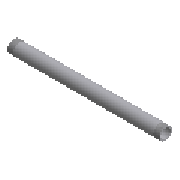
# Autodesk Inventor part: pipipe.1661247839230
Saved by Autodesk Inventor 2023 (Build 270158000, 158)
## iProperties
IsCustomPart: 1
Created: 2022-02-04
Material: Steel, Wrought
Description: Pipe
Document SubType Name: Modeling
Standard: ASME B36.10M
Designer: Mike
Standard Revision: 2004
Standards Organization: ANSI
Language: en-US
Size Designation: 1/2 - Schedule 30 - 4.25
Categories: <MemberInstance><Categories><Category DisplayName="Tube &amp; Pipe" InternalName="4347fa0f-2144-441d-94cd-e3e15c92b736" Mnemonic="TUBEANDPIPE"><CategoryParameter DisplayName="Number of Connections" InternalName="04e9c83a-9e20-4a98-a7e1-e8abe87a2846" Mnemonic="NUM_CONNECTIONS"/><CategoryParameter DisplayName="Angles" InternalName="0e0e4fa4-3bd3-4656-a22e-4e07c8c476f8" Mnemonic="ANGLES"><CategoryParameter DisplayName="Angle" InternalName="9188ad83-1b16-48b4-8b0a-76ce729dafa7" Mnemonic="ANGLE"/></CategoryParameter><CategoryParameter DisplayName="SKey" InternalName="3da84699-049a-4bc2-a65a-6696b77c242f" Mnemonic="SKEY"/><CategoryParameter DisplayName="ISOGEN Description" InternalName="7aa3ba45-b821-4467-8584-f9e6f15f2a7d" Mnemonic="ISOGENDESC"/><CategoryParameter DisplayName="ITEM-CODE" InternalName="99cc3b15-24d9-4d38-aac7-792cfbc57acf" Mnemonic="ITEMCODE"/><CategoryParameter DisplayName="NameOfComponent" InternalName="9c74ad13-48a1-45fe-b0f7-5447561f444a" Mnemonic="NAMEOFCOMPONENT"/><CategoryParameter DisplayName="InLineGroups" InternalName="d60be647-bc43-4c18-a13f-9fe4115f8e64" Mnemonic="INLINEGROUPS"/><Category DisplayName="Conduits" InternalName="0917448a-7f4d-4362-b21b-a60d05e1c56f" Mnemonic="CONDUITS"><CategoryParameter DisplayName="PipeLength" InternalName="84233622-ea40-4b53-b636-458d54f3a9e0" Mnemonic="PL"/><CategoryParameter DisplayName="Connections" InternalName="ef1b9597-584c-4227-9e47-647057e92f71" Mnemonic="PIPE_CONNECTIONS"><CategoryParameter DisplayName="Gender Neutral" InternalName="0135de5f-ee32-4593-8b66-ab45f5df415d" Mnemonic="NEUTRAL"/><CategoryParameter DisplayName="OuterDiameter" InternalName="082ea741-3dcf-4853-908c-481f2491b57d" Mnemonic="OD"/><CategoryParameter DisplayName="MinEngagement [% of MaxEngagement]" InternalName="3e1ca047-d004-446e-8b7d-e3d2ffcfa6ae" Mnemonic="MINENGAGEMENT"/><CategoryParameter DisplayName="FlipDirection" InternalName="6711cd9d-6b7e-47bf-b3fd-37395011a06e" Mnemonic="FLIPDIRECTION"/><CategoryParameter DisplayName="EndTreatment" InternalName="6bdd7eeb-ca9f-479f-914a-a6f58ba02ecf" Mnemonic="ENDTREATMENT"/><CategoryParameter DisplayName="NominalSize" InternalName="8d3dc73b-63e9-4bca-af78-1523b571a978" Mnemonic="NS"/><CategoryParameter DisplayName="InnerDiameter" InternalName="8f0e7e1d-0c1a-450d-a3ea-acf6fdc37b38" Mnemonic="ID"/><CategoryParameter DisplayName="Female" InternalName="91a68ca8-89f8-430e-94a7-98da7f5558a1" Mnemonic="FEMALE"/><CategoryParameter DisplayName="MaxEngagement" InternalName="ca99fb4d-bf82-4017-ae60-624d35c0ac37" Mnemonic="MAXENGAGEMENT"/><CategoryParameter DisplayName="DisplayName" InternalName="eb067ee5-9455-4a40-a436-ea6da7417161" Mnemonic="DISPLAYNAME"/><CategoryParameter DisplayName="Fixed" InternalName="fcf2b1e1-6728-4f9c-9e27-68dda4edbfa5" Mnemonic="FIXED"/><CategoryParameter DisplayName="ScheduleNumber" InternalName="fd9d4457-3734-4b7e-ad1f-37a31a426796" Mnemonic="SN"/></CategoryParameter><CategoryParameter DisplayName="Connections" InternalName="ef1b9597-584c-4227-9e47-647057e92f71" Mnemonic="PIPE_CONNECTIONS"><CategoryParameter DisplayName="Gender Neutral" InternalName="0135de5f-ee32-4593-8b66-ab45f5df415d" Mnemonic="NEUTRAL"/><CategoryParameter DisplayName="OuterDiameter" InternalName="082ea741-3dcf-4853-908c-481f2491b57d" Mnemonic="OD"/><CategoryParameter DisplayName="MinEngagement [% of MaxEngagement]" InternalName="3e1ca047-d004-446e-8b7d-e3d2ffcfa6ae" Mnemonic="MINENGAGEMENT"/><CategoryParameter DisplayName="FlipDirection" InternalName="6711cd9d-6b7e-47bf-b3fd-37395011a06e" Mnemonic="FLIPDIRECTION"/><CategoryParameter DisplayName="EndTreatment" InternalName="6bdd7eeb-ca9f-479f-914a-a6f58ba02ecf" Mnemonic="ENDTREATMENT"/><CategoryParameter DisplayName="NominalSize" InternalName="8d3dc73b-63e9-4bca-af78-1523b571a978" Mnemonic="NS"/><CategoryParameter DisplayName="InnerDiameter" InternalName="8f0e7e1d-0c1a-450d-a3ea-acf6fdc37b38" Mnemonic="ID"/><CategoryParameter DisplayName="Female" InternalName="91a68ca8-89f8-430e-94a7-98da7f5558a1" Mnemonic="FEMALE"/><CategoryParameter DisplayName="MaxEngagement" InternalName="ca99fb4d-bf82-4017-ae60-624d35c0ac37" Mnemonic="MAXENGAGEMENT"/><CategoryParameter DisplayName="DisplayName" InternalName="eb067ee5-9455-4a40-a436-ea6da7417161" Mnemonic="DISPLAYNAME"/><CategoryParameter DisplayName="Fixed" InternalName="fcf2b1e1-6728-4f9c-9e27-68dda4edbfa5" Mnemonic="FIXED"/><CategoryParameter DisplayName="ScheduleNumber" InternalName="fd9d4457-3734-4b7e-ad1f-37a31a426796" Mnemonic="SN"/></CategoryParameter><Category DisplayName="Pipes" InternalName="b7e6be6b-6eb8-4fff-9fa6-a2e6ed0c1528" Mnemonic="PIPES"/></Category></Category><Category DisplayName="DataType" InternalName="23b78d0f-2648-40c6-8793-ca6db495c9e8" Mnemonic="DATATYPE"><CategoryParameter DisplayName="DisplayName" InternalName="05415f3d-3907-474b-a020-eb9d644f4cf3" Mnemonic="DISPLAYNAME"/><CategoryParameter DisplayName="Standard" InternalName="0c0a119c-1e12-4c84-803f-101930972f5e" Mnemonic="STANDARD"/><CategoryParameter DisplayName="Description" InternalName="13903e3d-64b1-4950-80da-f627842ea37f" Mnemonic="DESCRIPTION"/><CategoryParameter DisplayName="Designation" InternalName="2675968c-4ce5-49e0-a4f5-552d29089031" Mnemonic="DESIGNATION"/><CategoryParameter DisplayName="Default Row" InternalName="2af9ec52-faaa-4026-b378-f9fa4afca842" Mnemonic="DEFAULTROW"/><CategoryParameter DisplayName="Folder Name" InternalName="3f06958e-8713-4116-9be7-ed6184ecc97b" Mnemonic="FOLDERNAME"/><CategoryParameter DisplayName="Revision Guid" InternalName="45a75005-10b1-4dfc-8d6d-dfe629f0b93c" Mnemonic="REVISIONGUID"/><CategoryParameter DisplayName="FileName" InternalName="8b46a4cc-9585-4fed-90c3-899f57e09a73" Mnemonic="FILENAME"/><CategoryParameter DisplayName="StdsOrg" InternalName="8f5914e1-4693-403f-8ab5-d37768198c9d" Mnemonic="STDSORG"/><CategoryParameter DisplayName="Family Version" InternalName="914462f6-6e19-4b14-ba84-155b9680b1d0" Mnemonic="FAMILYREVISION"/><CategoryParameter DisplayName="Standard Revision" InternalName="91d5a463-65c2-4fde-b823-3b7fea5e8e17" Mnemonic="STANDARDREVISION"/><CategoryParameter DisplayName="Member Revision" InternalName="a65d44b9-392f-4f4f-857b-e4b3d54996fe" Mnemonic="MEMBERREVISION"/><CategoryParameter DisplayName="ClipFormat" InternalName="bc51e27b-3422-4e78-93ef-cec197ddf230" Mnemonic="CLIPFORMAT"/><CategoryParameter DisplayName="Manufacturer" InternalName="cd6c7a72-a28a-4e50-99a9-2c7f4e13e5ad" Mnemonic="MANUFACTURER"/><CategoryParameter DisplayName="InternalName" InternalName="cf1d0246-76d9-4b4a-8305-fa0409afb5c1" Mnemonic="INTERNALNAME"/><CategoryParameter DisplayName="IsMetric" InternalName="e2385c5b-1ea4-4823-96a8-8de651266ec3" Mnemonic="ISMETRIC"/><Category DisplayName="Part" InternalName="c0e0b642-3bcb-4cc8-9e80-f96d35c4afa4" Mnemonic="PART"><CategoryParameter DisplayName="Part Number" InternalName="016b6077-bfbe-49bd-92c9-d8d59c39c941" Mnemonic="PARTNUMBER"/><CategoryParameter DisplayName="Stock Number" InternalName="4dba7c1c-e26c-444e-836c-b08b433409a8" Mnemonic="STOCKNUMBER"/><CategoryParameter DisplayName="Material Key" InternalName="5c9a8adb-dd2b-4535-b97f-0a94a95fe41f" Mnemonic="MATERIALKEY"/><CategoryParameter DisplayName="Material" InternalName="818a152a-d3c3-49ca-80ee-df7d91421b8e" Mnemonic="MATERIAL"/></Category></Category><Category DisplayName="LegacyMap" InternalName="dfeab48a-acc2-4514-a11c-1b8dc28c3d5f" Mnemonic="LEGACYMAP"><CategoryParameter DisplayName="CatalogID" InternalName="0da51c36-8fd3-4028-86cc-0c9c9e96136a" Mnemonic="CATALOGID"/><CategoryParameter DisplayName="FamilyID" InternalName="1c0b589c-8bbe-4e1e-80cf-07c0de42ac2a" Mnemonic="FAMILYID"/><CategoryParameter DisplayName="MemberID" InternalName="a368ea03-db8a-4d6e-962b-2aa46306b8f5" Mnemonic="MEMBERID"/></Category></Categories><FamilyTemplate Id="ASME B36.10M Pipe with Threaded Ends"><FamilyTemplateParameters><FamilyTemplateParameter ObjectType="kUserParameterObject" ValueType="xs:double" Id="1" ObjectReferenceKey="OD"/><FamilyTemplateParameter ObjectType="kUserParameterObject" ValueType="xs:double" Id="2" ObjectReferenceKey="t"/><FamilyTemplateParameter ObjectType="kUserParameterObject" ValueType="xs:double" Id="3" ObjectReferenceKey="PL"/><FamilyTemplateParameter ObjectType="kUserParameterObject" ValueType="xs:double" Id="4" ObjectReferenceKey="ID"/><FamilyTemplateParameter ObjectType="kUserParameterObject" ValueType="xs:double" Id="5" ObjectReferenceKey="L4"/><FamilyTemplateParameter ObjectType="kUserParameterObject" ValueType="xs:double" Id="6" ObjectReferenceKey="L"/><FamilyTemplateParameter ObjectType="kUserParameterObject" ValueType="xs:double" Id="7" ObjectReferenceKey="L2"/><FamilyTemplateParameter ObjectType="kUserParameterObject" ValueType="xs:double" Id="8" ObjectReferenceKey="D2"/><FamilyTemplateParameter ObjectType="kUserParameterObject" ValueType="xs:string" Id="120" ObjectReferenceKey="Size_Designation"/><FamilyTemplateParameter ObjectType="kUserParameterObject" ValueType="xs:double" Id="126" ObjectReferenceKey="PLmin"/><FamilyTemplateParameter ObjectType="kPropertyObject" ValueType="xs:string" Id="100" ObjectReferenceKey="{32853F0F-3444-11d1-9E93-0060B03C1CA6}" SubObjectId="52"/><FamilyTemplateParameter ObjectType="kPropertyObject" ValueType="xs:string" Id="105" ObjectReferenceKey="{32853F0F-3444-11d1-9E93-0060B03C1CA6}" SubObjectId="5"/><FamilyTemplateParameter ObjectType="kPartComponentDefinitionObject" ValueType="xs:string" Id="110" SubObjectId="Material"/><FamilyTemplateParameter ObjectType="kPropertyObject" ValueType="xs:string" Id="111" ObjectReferenceKey="{32853F0F-3444-11d1-9E93-0060B03C1CA6}" SubObjectId="55"/><FamilyTemplateParameter ObjectType="kThreadFeatureObject" ValueType="xs:structure" Id="300" ObjectReferenceKey="10020000100000000A230000000000008000000000000000" SubObjectId="ThreadInfo"><FamilyTemplateParameter ObjectType="" ValueType="xs:string" Id="301" SubObjectId="ThreadType"/><FamilyTemplateParameter ObjectType="" ValueType="xs:string" Id="302" SubObjectId="NominalDiameter"/></FamilyTemplateParameter><FamilyTemplateParameter ObjectType="kThreadFeatureObject" ValueType="xs:structure" Id="303" ObjectReferenceKey="100200001000000041230000000000008000000000000000" SubObjectId="ThreadInfo"><FamilyTemplateParameter ObjectType="" ValueType="xs:string" Id="304" SubObjectId="ThreadType"/><FamilyTemplateParameter ObjectType="" ValueType="xs:string" Id="305" SubObjectId="NominalDiameter"/></FamilyTemplateParameter></FamilyTemplateParameters></FamilyTemplate><CategoryParameterMap><ParamToTemplateMap><ParamToTemplate CategoryParameter="//CategoryParameter[@InternalName='d60be647-bc43-4c18-a13f-9fe4115f8e64']" ConstantValue="1"/><ParamToTemplate CategoryParameter="//CategoryParameter[@InternalName='04e9c83a-9e20-4a98-a7e1-e8abe87a2846']" ConstantValue="2"/><ParamToTemplate CategoryParameter="//CategoryParameter[@InternalName='0e0e4fa4-3bd3-4656-a22e-4e07c8c476f8']" ConstantValue=""/><ParamToTemplate CategoryParameter="//CategoryParameter[@InternalName='0e0e4fa4-3bd3-4656-a22e-4e07c8c476f8'][1]/CategoryParameter[@InternalName='9188ad83-1b16-48b4-8b0a-76ce729dafa7']" ConstantValue="3.14159265358979"/><ParamToTemplate CategoryParameter="//CategoryParameter[@InternalName='ef1b9597-584c-4227-9e47-647057e92f71'][1]/CategoryParameter[@InternalName='6711cd9d-6b7e-47bf-b3fd-37395011a06e']" ConstantValue="true"/><ParamToTemplate CategoryParameter="//CategoryParameter[@InternalName='ef1b9597-584c-4227-9e47-647057e92f71'][1]/CategoryParameter[@InternalName='eb067ee5-9455-4a40-a436-ea6da7417161']" ConstantValue="Connection1"/><ParamToTemplate CategoryParameter="//CategoryParameter[@InternalName='ef1b9597-584c-4227-9e47-647057e92f71'][1]/CategoryParameter[@InternalName='91a68ca8-89f8-430e-94a7-98da7f5558a1']" ConstantValue="false"/><ParamToTemplate CategoryParameter="//CategoryParameter[@InternalName='ef1b9597-584c-4227-9e47-647057e92f71'][1]/CategoryParameter[@InternalName='6bdd7eeb-ca9f-479f-914a-a6f58ba02ecf']" ConstantValue="Threaded"/><ParamToTemplate CategoryParameter="//CategoryParameter[@InternalName='ef1b9597-584c-4227-9e47-647057e92f71'][1]/CategoryParameter[@InternalName='fcf2b1e1-6728-4f9c-9e27-68dda4edbfa5']" ConstantValue="false"/><ParamToTemplate CategoryParameter="//CategoryParameter[@InternalName='ef1b9597-584c-4227-9e47-647057e92f71'][1]/CategoryParameter[@InternalName='ca99fb4d-bf82-4017-ae60-624d35c0ac37']" ConstantValue="0"/><ParamToTemplate CategoryParameter="//CategoryParameter[@InternalName='ef1b9597-584c-4227-9e47-647057e92f71'][1]/CategoryParameter[@InternalName='3e1ca047-d004-446e-8b7d-e3d2ffcfa6ae']" ConstantValue="20"/><ParamToTemplate CategoryParameter="//CategoryParameter[@InternalName='ef1b9597-584c-4227-9e47-647057e92f71'][2]/CategoryParameter[@InternalName='6711cd9d-6b7e-47bf-b3fd-37395011a06e']" ConstantValue="false"/><ParamToTemplate CategoryParameter="//CategoryParameter[@InternalName='ef1b9597-584c-4227-9e47-647057e92f71'][2]/CategoryParameter[@InternalName='eb067ee5-9455-4a40-a436-ea6da7417161']" ConstantValue="Connection2"/><ParamToTemplate CategoryParameter="//CategoryParameter[@InternalName='ef1b9597-584c-4227-9e47-647057e92f71'][2]/CategoryParameter[@InternalName='91a68ca8-89f8-430e-94a7-98da7f5558a1']" ConstantValue="false"/><ParamToTemplate CategoryParameter="//CategoryParameter[@InternalName='ef1b9597-584c-4227-9e47-647057e92f71'][2]/CategoryParameter[@InternalName='6bdd7eeb-ca9f-479f-914a-a6f58ba02ecf']" ConstantValue="Threaded"/><ParamToTemplate CategoryParameter="//CategoryParameter[@InternalName='ef1b9597-584c-4227-9e47-647057e92f71'][2]/CategoryParameter[@InternalName='fcf2b1e1-6728-4f9c-9e27-68dda4edbfa5']" ConstantValue="false"/><ParamToTemplate CategoryParameter="//CategoryParameter[@InternalName='ef1b9597-584c-4227-9e47-647057e92f71'][2]/CategoryParameter[@InternalName='ca99fb4d-bf82-4017-ae60-624d35c0ac37']" ConstantValue="0"/><ParamToTemplate CategoryParameter="//CategoryParameter[@InternalName='ef1b9597-584c-4227-9e47-647057e92f71'][2]/CategoryParameter[@InternalName='3e1ca047-d004-446e-8b7d-e3d2ffcfa6ae']" ConstantValue="20"/><ParamToTemplate CategoryParameter="//CategoryParameter[@InternalName='05415f3d-3907-474b-a020-eb9d644f4cf3']" ConstantValue="ASME B36.10M Pipe with Threaded Ends"/><ParamToTemplate CategoryParameter="//CategoryParameter[@InternalName='cf1d0246-76d9-4b4a-8305-fa0409afb5c1']" ConstantValue="4a736116-503a-44ad-a922-868ac6b46736"/><ParamToTemplate CategoryParameter="//CategoryParameter[@InternalName='3f06958e-8713-4116-9be7-ed6184ecc97b']" ConstantValue="ASME B36.10M(2)"/><ParamToTemplate CategoryParameter="//CategoryParameter[@InternalName='914462f6-6e19-4b14-ba84-155b9680b1d0']" ConstantValue="10"/><ParamToTemplate CategoryParameter="//CategoryParameter[@InternalName='13903e3d-64b1-4950-80da-f627842ea37f']" ConstantValue="Pipe"/><ParamToTemplate CategoryParameter="//CategoryParameter[@InternalName='8f5914e1-4693-403f-8ab5-d37768198c9d']" ConstantValue="ANSI"/><ParamToTemplate CategoryParameter="//CategoryParameter[@InternalName='0c0a119c-1e12-4c84-803f-101930972f5e']" ConstantValue="ASME B36.10M"/><ParamToTemplate CategoryParameter="//CategoryParameter[@InternalName='cd6c7a72-a28a-4e50-99a9-2c7f4e13e5ad']" TemplateParameter="104"/><ParamToTemplate CategoryParameter="//CategoryParameter[@InternalName='91d5a463-65c2-4fde-b823-3b7fea5e8e17']" ConstantValue="2004"/><ParamToTemplate CategoryParameter="//CategoryParameter[@InternalName='bc51e27b-3422-4e78-93ef-cec197ddf230']" ConstantValue="CF_INVENTOR.STDPARTS"/><ParamToTemplate CategoryParameter="//CategoryParameter[@InternalName='e2385c5b-1ea4-4823-96a8-8de651266ec3']" ConstantValue="false"/><ParamToTemplate CategoryParameter="//CategoryParameter[@InternalName='45a75005-10b1-4dfc-8d6d-dfe629f0b93c']" ConstantValue="1b3bb503-a999-4b6a-9afb-996931dc692f"/><ParamToTemplate CategoryParameter="//CategoryParameter[@InternalName='2af9ec52-faaa-4026-b378-f9fa4afca842']" ConstantValue="1"/><ParamToTemplate CategoryParameter="//CategoryParameter[@InternalName='0da51c36-8fd3-4028-86cc-0c9c9e96136a']" ConstantValue="4DA64A5D-C2A1-4499-9EC0-0CCCC70B216C"/><ParamToTemplate CategoryParameter="//CategoryParameter[@InternalName='1c0b589c-8bbe-4e1e-80cf-07c0de42ac2a']" ConstantValue="4a736116-503a-44ad-a922-868ac6b46736"/><ParamToTemplate CategoryParameter="//CategoryParameter[@InternalName='ef1b9597-584c-4227-9e47-647057e92f71'][1]/CategoryParameter[@InternalName='8d3dc73b-63e9-4bca-af78-1523b571a978']" ConstantValue="1/2"/><ParamToTemplate CategoryParameter="//CategoryParameter[@InternalName='ef1b9597-584c-4227-9e47-647057e92f71'][1]/CategoryParameter[@InternalName='fd9d4457-3734-4b7e-ad1f-37a31a426796']" ConstantValue="30"/><ParamToTemplate CategoryParameter="//CategoryParameter[@InternalName='ef1b9597-584c-4227-9e47-647057e92f71'][2]/CategoryParameter[@InternalName='8d3dc73b-63e9-4bca-af78-1523b571a978']" ConstantValue="1/2"/><ParamToTemplate CategoryParameter="//CategoryParameter[@InternalName='ef1b9597-584c-4227-9e47-647057e92f71'][2]/CategoryParameter[@InternalName='fd9d4457-3734-4b7e-ad1f-37a31a426796']" ConstantValue="30"/><ParamToTemplate CategoryParameter="//CategoryParameter[@InternalName='99cc3b15-24d9-4d38-aac7-792cfbc57acf']" ConstantValue=""/><ParamToTemplate CategoryParameter="//CategoryParameter[@InternalName='7aa3ba45-b821-4467-8584-f9e6f15f2a7d']" ConstantValue=""/><ParamToTemplate CategoryParameter="//CategoryParameter[@InternalName='8b46a4cc-9585-4fed-90c3-899f57e09a73']" ConstantValue="ASME B36.10M Pipe with Threaded Ends 1/2 - Schedule 30 - 4.25"/><ParamToTemplate CategoryParameter="//CategoryParameter[@InternalName='a65d44b9-392f-4f4f-857b-e4b3d54996fe']" ConstantValue="8A398487-0032-46BF-A39C-EAECB5F4E68C"/><ParamToTemplate CategoryParameter="//CategoryParameter[@InternalName='a368ea03-db8a-4d6e-962b-2aa46306b8f5']" ConstantValue="F72C0958-4233-4CEB-B2B5-21B09F7EE8A3"/><ParamToTemplate CategoryParameter="//CategoryParameter[@InternalName='2675968c-4ce5-49e0-a4f5-552d29089031']" TemplateParameter="100"/><ParamToTemplate CategoryParameter="//CategoryParameter[@InternalName='ef1b9597-584c-4227-9e47-647057e92f71'][1]/CategoryParameter[@InternalName='8f0e7e1d-0c1a-450d-a3ea-acf6fdc37b38']" TemplateParameter="4"/><ParamToTemplate CategoryParameter="//CategoryParameter[@InternalName='ef1b9597-584c-4227-9e47-647057e92f71'][2]/CategoryParameter[@InternalName='8f0e7e1d-0c1a-450d-a3ea-acf6fdc37b38']" TemplateParameter="4"/><ParamToTemplate CategoryParameter="//CategoryParameter[@InternalName='818a152a-d3c3-49ca-80ee-df7d91421b8e']" TemplateParameter="110"/><ParamToTemplate CategoryParameter="//CategoryParameter[@InternalName='ef1b9597-584c-4227-9e47-647057e92f71'][1]/CategoryParameter[@InternalName='082ea741-3dcf-4853-908c-481f2491b57d']" TemplateParameter="1"/><ParamToTemplate CategoryParameter="//CategoryParameter[@InternalName='ef1b9597-584c-4227-9e47-647057e92f71'][2]/CategoryParameter[@InternalName='082ea741-3dcf-4853-908c-481f2491b57d']" TemplateParameter="1"/><ParamToTemplate CategoryParameter="//CategoryParameter[@InternalName='016b6077-bfbe-49bd-92c9-d8d59c39c941']" TemplateParameter="105"/><ParamToTemplate CategoryParameter="//CategoryParameter[@InternalName='84233622-ea40-4b53-b636-458d54f3a9e0']" TemplateParameter="3"/><ParamToTemplate CategoryParameter="//CategoryParameter[@InternalName='4dba7c1c-e26c-444e-836c-b08b433409a8']" TemplateParameter="111"/></ParamToTemplateMap></CategoryParameterMap></MemberInstance>
Stock Number: ASME B36.10M Pipe with Threaded Ends 1/2 - Schedule 30
Density: 8.03 g/cm^3
Appearance: Steel
NAME: PIPING: ASME B36.10M Pipe with Threaded Ends
DATA: <meta><inlinegroups number="1" deflen="25.4"></inlinegroups><connections number="2"></connections><angles><a>3.14159265358979</a></angles></meta>
L: 6.710 in
PL: 6.710 in
Author: Mike
Autodesk Inventor part; units mm, degrees
ref_plane "YZ Plane" through (0, 0, 0) normal (1, 0, 0) x (0, 1, 0)
ref_plane "XZ Plane" through (0, 0, 0) normal (0, 1, 0) x (-1, 0, 0)
ref_plane "XY Plane" through (0, 0, 0) normal (0, 0, 1) x (1, 0, 0)
sketch "Sketch1" plane through (0, 0, 0) normal (0, 1, 0) x (-1, 0, 0)
  line L0 (0, 0) -> (-170.434, 0)
  line L1 (-170.434, 0) -> (-170.434, 8.255) construction
  line L2 (-170.434, 8.255) -> (-170.434, 10.3578)
  line L3 (-170.434, 10.3578) -> (-160.5072, 10.668)
  line L4 (-160.5072, 10.668) -> (-9.9268, 10.668)
  line L5 (-85.217, 0) -> (-85.217, 10.668) construction
  line L6 (-170.434, 8.255) -> (0, 8.255)
  line L7 (0, 0) -> (0, 8.255) construction
  line L8 (0, 8.255) -> (0, 10.3578)
  line L9 (0, 10.3578) -> (-9.9268, 10.668)
  line L10 (-156.878, 10.7814) -> (-156.878, 0) construction
  line L11 (-13.556, 10.7814) -> (-13.556, 0) construction
  line L12 (-160.5072, 10.668) -> (-156.878, 10.7814) construction
  line L13 (-160.5072, 10.668) -> (-160.5072, 0) construction
  line L14 (-9.9268, 10.668) -> (-13.556, 10.7814) construction
  line L15 (-9.9268, 10.668) -> (-9.9268, 0) construction
  dimension "d0" = 21.336
  dimension "d1" = 1.79
  dimension "d2" = 16.51
  dimension "d3" = 170.434
  dimension "d4" = 13.556
  dimension "d5" = 21.5628
  constraints: 32 end point, 7 perpendicular, 4 point on line, 3 collinear, 3 symmetric about line, 2 midpoint, 1 coincident, 1 horizontal, 1 parallel, 3 other
  measures "d0" diameter of L4 L0
  measures "d1" angle of L0 L3
  measures "d2" diameter of L6 L0
  measures "d3" distance of L0.start L0.end
  measures "d4" horizontal distance of L2.end L10.start
  measures "d5" diameter of L10.start L0
revolve "Revolution1" add sketch "Sketch1" angle 360 about axis through (0, 0, 0) along (1, 0, 0)
thread "Thread1" size "1/2" designation "1/2 - 14 NPT" standard "NPT" full length
thread "Thread2" size "1/2" designation "1/2 - 14 NPT" standard "NPT" full length
equation "\"d0\" = OD"
equation "\"d2\" = ID"
equation "\"d3\" = L"
equation "\"d4\" = L2"
equation "\"d5\" = D2"
equation "\"OD\" = 21.336"
equation "\"t\" = 2.413"
equation "\"L\" = PL"
equation "\"L4\" = 19.8501"
equation "\"ID\" = 16.51"
equation "\"PL\" = 170.434"
equation "\"D2\" = 21.56282"
equation "\"L2\" = 13.55598"
equation "\"Size_Designation\" = 1.2345"
equation "\"PLmin\" = 2 * L2"
body "Solid1"
